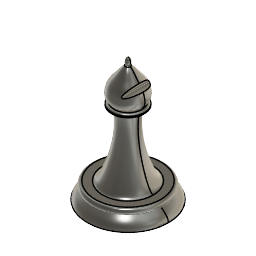
Nebun (Autodesk Fusion 360 design; units mm, degrees)
part number: 2026-03-27-16-39-54-698
Autodesk Fusion 360 part; units mm, degrees
sketch "Nebun" plane through (0, 0, 0) normal (0, 1, 0) x (1, 0, 0)
  line L0 (0, 0) -> (0, -46.4544)
  line L1 (0, -46.4544) -> (0, -45.1268) construction
  line L2 (0, -35) -> (0, -45.1268)
  arc A0 (0, -46.4544) -> (1, -46) centre (0, -45.1268) ccw
  line L3 (0, -32.0025) -> (3.4069, -32.0025)
  line L4 (3.4069, -32.0025) -> (5.4675, -32.0025)
  line L5 (9.9478, -6.4764) -> (0, -6.4764)
  line L6 (0, -49) -> (0, -46.4544)
  spline S0 degree 5 poles (0, -46.4544) (0.0754, -46.4311) (0.2198, -46.3948) (0.4172, -46.3713) (0.641, -46.4028) (0.8509, -46.5512) (0.9847, -46.8088) (1.036, -47.1672) (1.0017, -47.5979) (0.8824, -48.0528) (0.6792, -48.4775) (0.4497, -48.7506) (0.2397, -48.8993) (0.0827, -48.971) (0, -49) knots 0 0 0 0 0 0 0.1 0.2 0.3 0.4 0.5 0.6 0.7 0.8 0.9 1 1 1 1 1 1
  line L7 (0.2729, -48.9043) -> (-0.2729, -49.0957)
  line L8 (0, 0) -> (16, 0)
  line L9 (0, -6.4764) -> (12.9366, -6.4764)
  line L10 (12.9366, -4.0764) -> (0, -4.0764)
  line L11 (0, -4.0764) -> (0, -6.4764)
  arc A1 (12.9366, -6.4764) -> (14.1366, -5.2855) centre (12.9366, -5.2764) ccw
  arc A2 (14.1366, -5.2855) -> (12.9366, -4.0764) centre (12.9366, -5.2764) ccw
  spline S1 degree 5 poles (12.9366, -4.0764) (13.1271, -3.9343) (13.5002, -3.6476) (14.0361, -3.2102) (14.7, -2.6114) (15.4041, -1.8243) (15.8034, -1.1441) (15.9642, -0.5913) (16, -0.2008) (16, 0) knots 0 0 0 0 0 0 0.2 0.4 0.6 0.8 1 1 1 1 1 1
  line L12 (16, -0.463) -> (16, 0.463)
  line L13 (0, -33.5564) -> (5.4675, -33.5564)
  spline S2 degree 5 poles (1, -46) (1.0428, -45.9606) (1.127, -45.8825) (1.2496, -45.7674) (1.4055, -45.6178) (1.5877, -45.4373) (1.7578, -45.2628) (1.917, -45.0931) (2.0669, -44.9266) (2.2103, -44.7605) (2.3506, -44.5914) (2.4916, -44.4159) (2.6365, -44.2312) (2.7873, -44.0357) (2.9446, -43.8302) (3.107, -43.6175) (3.2717, -43.4017) (3.4359, -43.1875) (3.5967, -42.9791) (3.7521, -42.7796) (3.9018, -42.5897) (4.047, -42.4082) (4.1899, -42.2323) (4.3327, -42.0587) (4.4778, -41.884) (4.6264, -41.705) (4.7787, -41.5199) (4.9342, -41.3276) (5.0913, -41.128) (5.2481, -40.9217) (5.402, -40.7106) (5.5503, -40.4973) (5.6899, -40.285) (5.8185, -40.0766) (5.9341, -39.8743) (6.0357, -39.6789) (6.1236, -39.4894) (6.1993, -39.3029) (6.2652, -39.1158) (6.3237, -38.9245) (6.3773, -38.726) (6.4282, -38.519) (6.4776, -38.3035) (6.5263, -38.081) (6.5739, -37.8538) (6.619, -37.6253) (6.6591, -37.3992) (6.691, -37.1796) (6.712, -36.9697) (6.7203, -36.7711) (6.7158, -36.5835) (6.701, -36.4038) (6.6795, -36.2273) (6.6541, -36.05) (6.6259, -35.8693) (6.5924, -35.686) (6.5483, -35.5037) (6.4876, -35.3265) (6.4054, -35.1579) (6.3, -34.9985) (6.1733, -34.8459) (6.0294, -34.6971) (5.8729, -34.5499) (5.7084, -34.4052) (5.5382, -34.2692) (5.363, -34.1508) (5.1825, -34.0577) (4.9957, -33.9928) (4.8019, -33.95) (4.6011, -33.911) (4.3938, -33.8513) (4.2232, -33.7669) (4.0929, -33.6741) (4.0051, -33.598) (3.9609, -33.5564) knots 0 0 0 0 0 0 0.01428571 0.02857143 0.04285714 0.05714286 0.07142857 0.08571429 0.1 0.11428571 0.12857143 0.14285714 0.15714286 0.17142857 0.18571429 0.2 0.21428571 0.22857143 0.24285714 0.25714286 0.27142857 0.28571429 0.3 0.31428571 0.32857143 0.34285714 0.35714286 0.37142857 0.38571429 0.4 0.41428571 0.42857143 0.44285714 0.45714286 0.47142857 0.48571429 0.5 0.51428571 0.52857143 0.54285714 0.55714286 0.57142857 0.58571429 0.6 0.61428571 0.62857143 0.64285714 0.65714286 0.67142857 0.68571429 0.7 0.71428571 0.72857143 0.74285714 0.75714286 0.77142857 0.78571429 0.8 0.81428571 0.82857143 0.84285714 0.85714286 0.87142857 0.88571429 0.9 0.91428571 0.92857143 0.94285714 0.95714286 0.97142857 0.98571429 1 1 1 1 1 1
  line L14 (5.5565, -35.059) -> (2.3653, -32.0538)
  line L15 (6.4675, -32.5564) -> (6.4675, -33.0025)
  arc A3 (5.4675, -33.5564) -> (6.4675, -32.5564) centre (5.4675, -32.5564) ccw
  arc A4 (6.4675, -33.0025) -> (5.4675, -32.0025) centre (5.4675, -33.0025) ccw
  spline S3 degree 5 poles (4.4372, -32.0025) (4.3926, -31.7636) (4.3089, -31.2754) (4.1994, -30.5122) (4.0855, -29.4321) (3.9996, -27.9741) (3.9765, -26.4008) (4.0266, -24.702) (4.1657, -22.8634) (4.4123, -20.8737) (4.7831, -18.7344) (5.2885, -16.4691) (5.9279, -14.1341) (6.6841, -11.8299) (7.5173, -9.7149) (8.3754, -7.9746) (9.04, -7.0247) (9.5079, -6.6229) (9.8038, -6.501) (9.9478, -6.4764) knots 0 0 0 0 0 0 0.066667 0.133333 0.2 0.266667 0.333333 0.4 0.466667 0.533333 0.6 0.666667 0.733333 0.8 0.866667 0.933333 1 1 1 1 1 1
  line L16 (8.9423, -6.6477) -> (10.9532, -6.3052)
  spline S4 degree 5 poles (4.4165, -41.9579) (4.2811, -41.7738) (4.0247, -41.4179) (3.6836, -40.9207) (3.317, -40.3323) (3.0158, -39.7297) (2.8861, -39.2721) (2.9422, -38.9716) (3.1927, -38.8355) (3.6309, -38.8581) (4.2431, -39.0278) (4.8608, -39.2718) (5.3915, -39.5118) (5.7748, -39.6967) (5.9738, -39.7954) knots 0 0 0 0 0 0 0.1 0.2 0.3 0.4 0.5 0.6 0.7 0.8 0.9 1 1 1 1 1 1
  point P0 (9.9942, -32.0025)
  point P1 (9.994, -33.0025)
  point P2 (2, -45)
  point P3 (2.7357, -44.1024)
  point P4 (3.6547, -42.9048)
  point P5 (4.4165, -41.9579)
  point P6 (5.2422, -40.9275)
  point P7 (5.9738, -39.7954)
  point P8 (6.3277, -38.9044)
  point P9 (6.5754, -37.8427)
  point P10 (6.717, -36.7809)
  point P11 (6.6462, -36.0022)
  point P12 (6.4339, -35.2236)
  point P13 (5.8322, -34.5157)
  point P14 (5, -34)
  point P15 (4, -26)
  point P16 (6, -14)
  point P17 (1, -47)
  point P18 (3, -39)
  dimension "d8" = 1
  dimension "d11" = 16
  dimension "d12" = 1.2
  dimension "d14" = 1
  dimension "d21" = 49
  constraint coincident L0.start L8.start
  constraint parallel L0 L1
  constraint vertical L2
  constraint coincident L1.end L2.end
  constraint coincident L0 L3.start
  constraint perpendicular L0 L3
  constraint parallel L3 L4
  constraint coincident P0 L4
  constraint coincident L0 L5.end
  constraint perpendicular L0 L5
  constraint coincident L4 S3.start
  constraint coincident L6.start S0.end
  constraint parallel L1 L6
  constraint midpoint L6.start L7
  constraint perpendicular L0 L8
  constraint horizontal L9
  constraint horizontal L10
  constraint vertical L11
  constraint tangent L9 A1
  constraint tangent L10 A2
  constraint equal A1 A2
  constraint midpoint L8.end L12
  constraint coincident L0 L13.start
  constraint perpendicular L0 L13
  constraint coincident L13 S2.end
  constraint midpoint S2.end L14
  constraint perpendicular L4 L15
  constraint tangent L13 A3
  constraint tangent L15 A3
  constraint tangent L4 A4
  constraint tangent L15 A4
  constraint equal A3 A4
  constraint midpoint L5.start L16
  constraint coincident P5 S4.start
  constraint coincident P7 S4.end
  measures "d8" distance of P0 P1
  measures "d11" distance of L0.start L8.end
  measures "d12" radius of A1
  measures "d14" radius of A3
  measures "d21" distance of L0.start L6.start
revolve "Revolve2" add sketch "Nebun" angle 360 about axis through (0, 0, 0) along (0, 0, 1)
extrude "Extrude1" cut sketch "Nebun" along normal blind 6 contours S2 S4
extrude "Extrude2" cut sketch "Nebun" against normal blind 6 contours S2 S4
named bodies: "Nebun"
